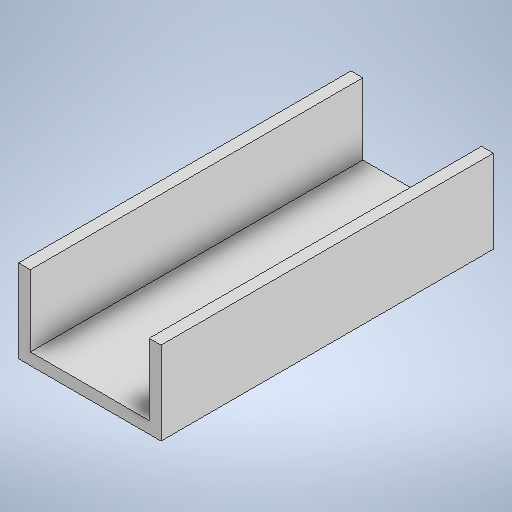
# Autodesk Inventor part: track z2229
Saved by Autodesk Inventor 2025.3 (Build 293356000, 356)
## iProperties
Created: 2026-04-19
Part Number: track z2229
Material: Generic
Document SubType Name: Modeling
Designer: kamal
Density: 1 g/cm^3
Appearance: Default
Author: kamal
Autodesk Inventor part; units mm, degrees
ref_plane "YZ Plane" through (0, 0, 0) normal (1, 0, 0) x (0, 1, 0)
ref_plane "XZ Plane" through (0, 0, 0) normal (0, 1, 0) x (-1, 0, 0)
ref_plane "XY Plane" through (0, 0, 0) normal (0, 0, 1) x (1, 0, 0)
sketch "Sketch1" plane through (0, 0, 0) normal (0, 0, 1) x (1, 0, 0)
  line L0 (25, 0) -> (-25, 0)
  line L1 (-25, 0) -> (-25, 30)
  line L2 (-25, 30) -> (-30, 30)
  line L3 (-30, 30) -> (-30, -5)
  line L4 (-30, -5) -> (30, -5)
  line L5 (30, -5) -> (30, 30)
  line L6 (30, 30) -> (25, 30)
  line L7 (25, 30) -> (25, 0)
  point P0 (0, 0)
  dimension "d0" = 50
  dimension "d1" = 30
  dimension "d2" = 5
  dimension "d3" = 35
  dimension "d4" = 60
  dimension "d5" = 35
  dimension "d6" = 5
  constraints: 16 end point, 2 horizontal, 2 perpendicular, 2 point on line, 1 midpoint, 1 vertical
  measures "d0" distance of L0.start L0.end
  measures "d1" distance of L0.end L1.end
  measures "d2" distance of L1.end L2.end
  measures "d3" distance of L2.end L3.end
  measures "d4" distance of L3.end L4.end
  measures "d5" distance of L4.end L5.end
  measures "d6" distance of L5.end L6.end
extrude "Extrusion1" add sketch "Sketch1" along normal blind 140
body "Solid1"
